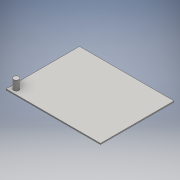
# Autodesk Inventor part: protoboard
Saved by Autodesk Inventor 2016 (Build 200138000, 138)
## iProperties
Created: 2015-09-18
Part Number: protoboard
Material: Generic
Document SubType Name: Modeling
Designer: Erin
Density: 1 g/cm^3
Appearance: Default
Author: Erin
Autodesk Inventor part; units mm, degrees
ref_plane "YZ Plane" through (0, 0, 0) normal (1, 0, 0) x (0, 1, 0)
ref_plane "XZ Plane" through (0, 0, 0) normal (0, 1, 0) x (-1, 0, 0)
ref_plane "XY Plane" through (0, 0, 0) normal (0, 0, 1) x (1, 0, 0)
sketch "Sketch1" plane through (0, 0, 0) normal (0, 0, 1) x (1, 0, 0)
  line L0 (-47.2018, -34.166) -> (42.7982, -34.166)
  line L1 (42.7982, -34.166) -> (42.7982, 35.834)
  line L2 (42.7982, 35.834) -> (-47.2018, 35.834)
  line L3 (-47.2018, 35.834) -> (-47.2018, -34.166)
  circle A0 centre (-42.2305, -29.3992) radius 2.5544
  point P0 (0, 0)
  dimension "d0" = 90
  dimension "d1" = 70
  constraints: 8 end point, 2 parallel, 1 centre point, 1 horizontal, 1 perpendicular
  measures "d0" distance of L2.end L1.end
  measures "d1" distance of L1.end L0.end
extrude "Extrusion1" add sketch "Sketch1" along normal blind 1 contours L3 L2 L1 L0 | A0
extrude "Extrusion2" add sketch "Sketch1" along normal blind 10 contours A0
body "Solid1"
